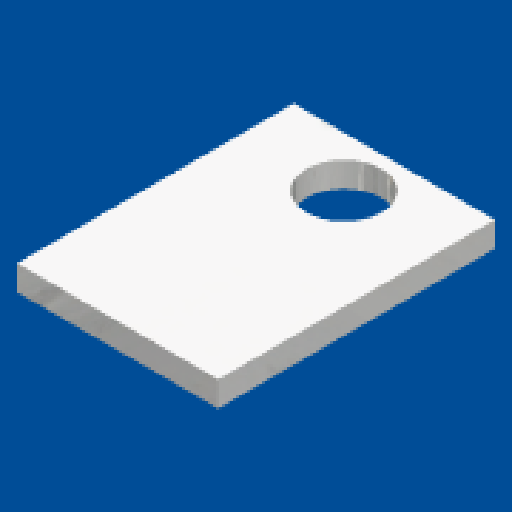
# Autodesk Inventor part: basePlatform
Saved by Autodesk Inventor 2023 (Build 270158030, 158C)
## iProperties
Created: 2023-03-03
Part Number: basePlatform
Material: Aluminum 6061
Document SubType Name: Modeling
Designer: kumpu
Density: 2.7 g/cm^3
Appearance: Aluminum - Dark
Mass: 447.602 g
Surface Area: 337.56 cm^2
Volume: 165.779 cm^3
Author: kumpu
Autodesk Inventor part; units mm, degrees
ref_plane "YZ Plane" through (0, 0, 0) normal (1, 0, 0) x (0, 1, 0)
ref_plane "XZ Plane" through (0, 0, 0) normal (0, 1, 0) x (-1, 0, 0)
ref_plane "XY Plane" through (0, 0, 0) normal (0, 0, 1) x (1, 0, 0)
sketch "Sketch1" plane through (0, 0, 0) normal (0, 1, 0) x (-1, 0, 0)
  circle A0 centre (0, 0) radius 19.05
  line L0 (-50.8, 107.95) -> (50.8, 107.95)
  line L1 (50.8, 107.95) -> (50.8, -31.75)
  line L2 (50.8, -31.75) -> (-50.8, -31.75)
  line L3 (-50.8, -31.75) -> (-50.8, 107.95)
  line L4 (-50.8, 107.95) -> (50.8, -31.75) construction
  line L5 (50.8, 107.95) -> (-50.8, -31.75) construction
  line L6 (0, 0) -> (0, 38.1) construction
  dimension "d0" = 38.1
  dimension "d1" = 31.75
  dimension "d2" = 101.6
  dimension "d3" = 139.7
  constraints: 14 end point, 2 midpoint, 2 parallel, 1 centre point, 1 coincident, 1 horizontal, 1 perpendicular, 1 vertical
  measures "d0" diameter of A0
  measures "d1" distance from line of point (0, 0) L2
  measures "d2" distance of L1.end L2.end
  measures "d3" distance of L0.end L1.end
extrude "Extrusion1" add sketch "Sketch1" along normal blind 12.7
body "Solid1"
